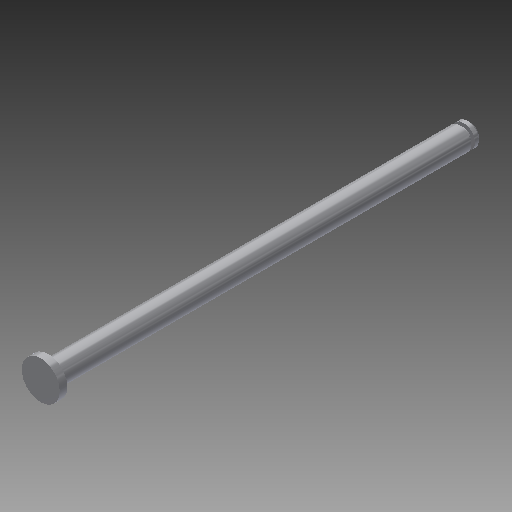
# Autodesk Inventor part: Axle
Saved by Autodesk Inventor 2019 (Build 230136000, 136)
## iProperties
Created: 2013-01-20
Part Number: Axle
Material: Aluminum 6061
Document SubType Name: Modeling
Designer: banachd
Density: 1 g/cm^3
Description: 3 mm DIA x 55.5 mm
Appearance: Aluminum - Flat
Author: banachd
Autodesk Inventor part; units mm, degrees
ref_plane "YZ Plane" through (0, 0, 0) normal (1, 0, 0) x (0, 1, 0)
ref_plane "XZ Plane" through (0, 0, 0) normal (0, 1, 0) x (-1, 0, 0)
ref_plane "XY Plane" through (0, 0, 0) normal (0, 0, 1) x (1, 0, 0)
sketch "Sketch1" plane through (0, 0, 0) normal (0, 0, 1) x (1, 0, 0)
  circle A0 centre (0, 0) radius 1.5
  dimension "d0" = 3
  constraints: 1 centre point, 1 coincident
  measures "d0" diameter of A0
extrude "Extrusion1" add sketch "Sketch1" along normal blind 55.5
sketch "Sketch2" plane through (0, 0, 55.5) normal (0, 0, 1) x (1, 0, 0)
  circle A0 centre (0, 0) radius 1.5 projected
  circle A1 centre (0, 0) radius 2.5
  dimension "d3" = 5
  constraints: 1 centre point, 1 coincident
  measures "d3" diameter of A1
extrude "Extrusion2" add sketch "Sketch2" along normal blind 1 contours A0 | A1
sketch "Sketch3" plane through (0, 0, 0) normal (1, 0, 0) x (0, 1, 0)
  line L0 (-1.5, 55.5) -> (-2.5, 55.5) projected
  line L1 (-2.5, 55.5) -> (-2.5, 56.5) projected
  line L2 (-2.5, 56.5) -> (2.5, 56.5) projected
  line L3 (2.5, 56.5) -> (2.5, 55.5) projected
  line L4 (2.5, 55.5) -> (1.5, 55.5) projected
  line L5 (1.5, 55.5) -> (1.5, 0) projected
  line L6 (1.5, 0) -> (-1.5, 0) projected
  line L7 (-1.5, 0) -> (-1.5, 55.5) projected
  line L8 (1.5, 1.5) -> (1, 1.5)
  line L9 (1, 1.5) -> (1, 1)
  line L10 (1, 1) -> (1.5, 1)
  line L11 (1.5, 1) -> (1.5, 1.5)
  line L12 (0, -11.4) -> (0, 68.4) projected
  point P0 (0, 0)
  dimension "d6" = 54
  dimension "d7" = 0.5
  dimension "d8" = 0.5
  constraints: 8 end point, 2 parallel, 1 horizontal, 1 perpendicular, 1 point on line
  measures "d6" distance from line of L4.end L8
  measures "d7" distance between parallel lines of L10 L8
  measures "d8" distance of L9.end L10.end
revolve "Revolution1" cut sketch "Sketch3" angle 360 about axis through (0, 0, -10) along (0, 0, 1) contours L10 L9 L8 L5
chamfer "Chamfer1" distance 0.5 angle 45 1 edges at (-1.5, 0, 0)
body "Solid1"
